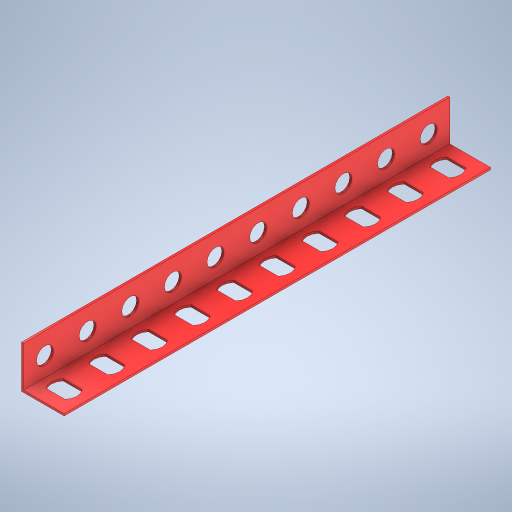
# Autodesk Inventor part: 1027
Saved by Autodesk Inventor 2024 (Build 280153000, 153)
## iProperties
Created: 2024-09-20
Part Number: 1027
Material: Všeobecné
Document SubType Name: Modeling
Designer: Student
Density: 1 g/cm^3
Appearance: Světle červená
Author: Student
Autodesk Inventor part; units mm, degrees
ref_plane "YZ Plane" through (0, 0, 0) normal (1, 0, 0) x (0, 1, 0)
ref_plane "XZ Plane" through (0, 0, 0) normal (0, 1, 0) x (-1, 0, 0)
ref_plane "XY Plane" through (0, 0, 0) normal (0, 0, 1) x (1, 0, 0)
sketch "Náčrt1" plane through (0, 0, 0) normal (0, 0, 1) x (1, 0, 0)
  line L0 (1.3202, 0) -> (0, 0)
  line L1 (0, 0) -> (0, 10)
  line L2 (0, 10) -> (0.5, 10)
  line L3 (0.5, 10) -> (0.5, 0.5)
  line L4 (0.5, 0.5) -> (10, 0.5)
  line L5 (10, 0.5) -> (10, 0)
  line L6 (10, 0) -> (1.3202, 0)
  point P0 (10, 0.25)
  point P1 (0.25, 10)
  dimension "d0" = 0.5
  dimension "d1" = 0.5
  dimension "d2" = 10
  dimension "d3" = 10
  constraints: 14 end point, 5 perpendicular, 2 midpoint, 1 collinear, 1 horizontal, 1 point on line
  measures "d0" distance between parallel lines of L1 L3
  measures "d1" distance between parallel lines of L4 L6
  measures "d2" distance from line of L1 point (10, 0.25)
  measures "d3" distance from line of point (0.25, 10) L0
extrude "Vysunutí1" add sketch "Náčrt1" along normal blind 100
sketch "Náčrt2" plane through (0.5, 0.5, 0) normal (0, 1, 0) x (1, 0, 0)
  line L0 (9.5, 0) -> (0, 0) projected
  line L1 (9.5, 0) -> (9.5, -100) projected
  line L2 (2.2639, -3) -> (6.7361, -3)
  line L3 (2.2639, -7) -> (6.7361, -7)
  arc A0 (2.2639, -3) -> (2.2639, -7) centre (4.5, -5) ccw
  arc A1 (6.7361, -7) -> (6.7361, -3) centre (4.5, -5) ccw
  point P0 (-0.5, 0)
  point P1 (4.8669, -7)
  dimension "d7" = 5
  dimension "d8" = 5
  dimension "d9" = 2
  dimension "d10" = 4
  constraints: 4 end point, 4 point on circle, 2 centre point, 1 horizontal, 1 perpendicular, 1 point on line
  measures "d7" distance from line of L0 A0.centre
  measures "d8" distance from line of L1 A0.centre
  measures "d9" distance from line of A0.centre L2
  measures "d10" distance from line of point (4.867, -7) L2
extrude "Vysunutí2" cut sketch "Náčrt2" against normal through all
pattern_linear "Obdélníkové pole1" count 10 spacing 10 along (0, 0, 1) of "Vysunutí2"
sketch "Náčrt4" plane through (0.5, 0.5, 0) normal (1, 0, 0) x (0, 0, -1)
  line L0 (0, 0) -> (0, 9.5) projected
  line L1 (0, 9.5) -> (-100, 9.5) projected
  line L2 (-100, 0) -> (-100, 9.5) projected
  circle A0 centre (-5, 4.5) radius 2
  point P0 (0, -0.5)
  point P1 (-5, 9.5)
  point P2 (0, 4.5)
  point P3 (-100, 4.5)
  point P4 (-95, 9.5)
  dimension "d30" = 4
  constraints: 4 point on line, 1 centre point
  measures "d30" diameter of A0
extrude "Vysunutí4" cut sketch "Náčrt4" against normal blind 10
sketch "Náčrt5" plane through (0.5, 0.5, 100) normal (1, 0, 0) x (0, 0, -1)
  circle A0 centre (5, 4.5) radius 2
  line L0 (100, 9.5) -> (0, 9.5) projected
  line L1 (0, 0) -> (0, 9.5) projected
  point P0 (100, -0.5)
  point P1 (95, 9.5)
  point P2 (5, 9.5)
  point P3 (0, 4.5)
  dimension "d33" = 4
  dimension "d34" = 5
  dimension "d35" = 5
  constraints: 1 centre point
  measures "d33" diameter of A0
  measures "d34" distance from line of L0 A0.centre
  measures "d35" distance from line of L1 A0.centre
extrude "Vysunutí5" cut sketch "Náčrt5" against normal blind 10
pattern_linear "Obdélníkové pole3" count 10 spacing 10 along (0, 0, -1) of "Vysunutí5"
